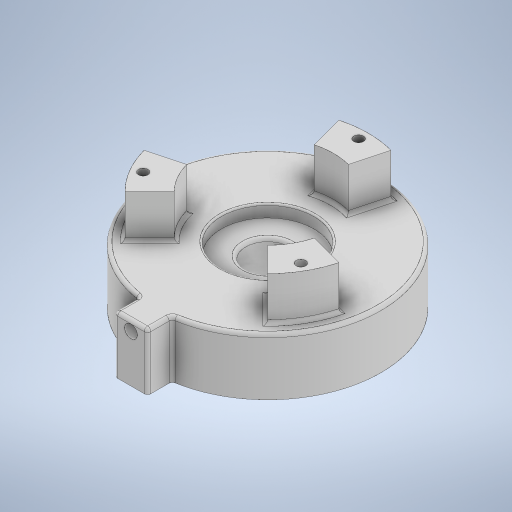
# Autodesk Inventor part: Dewar-YDS-3-Adapter
Saved by Autodesk Inventor 2023 (Build 270158000, 158)
## iProperties
Created: 2024-06-03
Part Number: Dewar-YDS-3-Adapter
Material: Generic
Document SubType Name: Modeling
Designer: incep
Density: 1 g/cm^3
Appearance: Default
Author: incep
Autodesk Inventor part; units mm, degrees
ref_plane "YZ Plane" through (0, 0, 0) normal (1, 0, 0) x (0, 1, 0)
ref_plane "XZ Plane" through (0, 0, 0) normal (0, 1, 0) x (-1, 0, 0)
sketch "Sketch1" plane through (0, 0, 0) normal (0, 1, 0) x (-1, 0, 0)
  circle A0 centre (0, 0) radius 38.75 construction
  circle A1 centre (0, 0) radius 39.25
  circle A2 centre (0, 0) radius 60.865
  circle A3 centre (0, 0) radius 60.865 construction
  dimension "d0" = 77.5
  dimension "d1" = 0.5
  dimension "d19" = 121.73
  constraints: 4 centre point, 2 coincident, 1 concentric
  measures "d0" diameter of A0
  measures "d1" radial gap between concentric circles of A0 A1
  measures "d19" diameter of A3
extrude "Extrusion1" add sketch "Sketch1" along normal blind 21
sketch "Sketch2" plane through (0, 21, 0) normal (0, 1, 0) x (1, 0, 0)
  circle A0 centre (0, 0) radius 60.865 projected
extrude "Extrusion2" add sketch "Sketch2" along normal blind 6
sketch "Sketch3" plane through (0, 27, 0) normal (0, 1, 0) x (1, 0, 0)
  circle A0 centre (0, 0) radius 12.7 construction
  circle A1 centre (0, 0) radius 13.2
  dimension "d7" = 25.4
  dimension "d8" = 0.5
  constraints: 2 centre point, 1 coincident
  measures "d7" diameter of A0
  measures "d8" radial gap between concentric circles of A0 A1
extrude "Extrusion3" cut sketch "Sketch3" against normal blind 10
sketch "Sketch4" plane through (0, 21, 0) normal (0, -1, 0) x (1, 0, 0)
  circle A0 centre (0, 0) radius 13.2 projected
  circle A1 centre (0, 0) radius 25 construction
  circle A2 centre (0, 0) radius 24.5
  dimension "d11" = 50
  dimension "d12" = 0.5
  constraints: 2 centre point, 1 coincident
  measures "d11" diameter of A1
  measures "d12" radial gap between concentric circles of A1 A2
extrude "Extrusion4" add sketch "Sketch4" along normal up to surface (21 mm away)
sketch "Sketch5" plane through (0, 27, 0) normal (0, 1, 0) x (1, 0, 0)
  circle A0 centre (0, 0) radius 60.865 projected
  circle A1 centre (0, 0) radius 27.45 construction
  circle A2 centre (0, 0) radius 27.95
  dimension "d15" = 54.9
  dimension "d16" = 0.5
  constraints: 2 centre point, 1 coincident
  measures "d15" diameter of A1
  measures "d16" radial gap between concentric circles of A1 A2
extrude "Extrusion5" add sketch "Sketch5" along normal blind 7.5
sketch "Sketch6" plane through (0, 34.5, 0) normal (0, 1, 0) x (1, 0, 0)
  circle A0 centre (0, 0) radius 27.95 construction
  circle A1 centre (0, 0) radius 55 construction
  circle A2 centre (0, 55) radius 2.9
  circle A3 centre (0, 0) radius 60.865 projected
  circle A4 centre (0, 0) radius 39.85
  line L0 (0, 0) -> (15.753, 58.7911)
  line L1 (0, 55) -> (0, 0) construction
  line L2 (0, 0) -> (-15.753, 58.7911)
  point P0 (-10.3139, 38.4921)
  point P1 (10.3139, 38.4921)
  dimension "d20" = 110
  dimension "d21" = 5.8
  dimension "d23" = 79.7
  dimension "d24" = 15
  constraints: 6 end point, 2 centre point, 2 vertical alignment, 1 coincident, 1 symmetric about line, 1 vertical, 4 other
  measures "d21" diameter of A2
  measures "d23" diameter of A4
  measures "d24" angle of L1 L0
extrude "Extrusion6" add sketch "Sketch6" along normal blind 26.1 contours L0 A4 L2 A3 picked at (9.5449, 50.3118)
pattern_circular "Circular Pattern1" count 3 over 360 about axis through (0, -10, 0) along (0, 1, 0) of "Extrusion6"
fillet "Fillet2" radius 1 1 edges at (-27.95, 34.5, 0)
sketch "Sketch7" plane through (0, 0, 0) normal (1, 0, 0) x (0, 1, 0)
  line L0 (6.175, 11.9062) -> (3, 11.9062)
  line L1 (3, 11.9062) -> (3, 15.0812)
  line L2 (3, 15.0812) -> (6.175, 15.0813)
  line L3 (6.175, 15.0813) -> (6.175, 11.9062)
  line L4 (27, -27.95) -> (27, 27.95) projected
  line L5 (-12.12, 0) -> (72.72, 0) projected
  line L6 (0, -13.2) -> (0, 13.2) projected
  line L7 (0, 24.5) -> (0, -24.5) projected
  point P0 (0, 0)
  point P1 (27, -16.2)
  point P2 (27, 16.2)
  dimension "d35" = 3.175
  dimension "d36" = 3.175
  dimension "d42" = 3
  dimension "d43" = 15.0813
  constraints: 8 end point, 2 parallel, 1 horizontal, 1 perpendicular
  measures "d35" distance of L0.start L0.end
  measures "d36" distance of L2.end L0.start
  measures "d42" distance between parallel lines of L1 L6
  measures "d43" distance from line of point (0, 0) L2
revolve "Revolution1" cut sketch "Sketch7" angle 360 about axis through (0, -10, 0) along (0, 1, 0)
sketch "Sketch9" plane through (0, 0, 0) normal (0, -1, 0) x (1, 0, 0)
  circle A0 centre (0, 0) radius 49.25
  circle A1 centre (0, 0) radius 39.25 projected
  circle A2 centre (0, 0) radius 60.865 projected
  circle A3 centre (0, 0) radius 13.2 projected
  line L0 (0, 0) -> (15.753, -58.7911)
  line L1 (0, 0) -> (0, -60.865) construction
  line L2 (0, 0) -> (-15.753, -58.7911)
  line L3 (0, 0) -> (52.7106, 30.4325) construction
  line L4 (0, 0) -> (52.7106, 30.4325)
  line L5 (0, 0) -> (58.7911, 15.753)
  point P0 (47.5718, 12.7468)
  point P1 (12.7468, -47.5718)
  dimension "d44" = 10
  dimension "d45" = 15
  dimension "d46" = 120
  dimension "d47" = 15
  constraints: 12 end point, 5 point on circle, 1 centre point, 1 coincident, 1 symmetric about line, 1 vertical
  measures "d44" radial gap between concentric circles of A0 A1
  measures "d45" angle of L0 L1
  measures "d46" angle of L1 L3
  measures "d47" angle of L5 L3
extrude "Extrusion8" cut sketch "Sketch9" against normal up to surface (34.5 mm away) contours A0 L5 A2 L0
pattern_circular "Circular Pattern2" count 3 over 360 about axis through (0, -10, 0) along (0, 1, 0) of "Extrusion8"
sketch "Sketch10" plane through (0, 0, 0) normal (0, -1, 0) x (1, 0, 0)
  circle A0 centre (0, 0) radius 68.5
  line L0 (43.0381, 43.0381) -> (34.825, 34.825) projected
  arc A1 (34.825, 34.825) -> (-34.825, 34.825) centre (0, 0) ccw projected
  line L1 (-34.825, 34.825) -> (-43.0381, 43.0381) projected
  arc A2 (-43.0381, 43.0381) -> (-58.7911, 15.753) centre (0, 0) ccw projected
  line L2 (-58.7911, 15.753) -> (-47.5718, 12.7468) projected
  arc A3 (-47.5718, 12.7468) -> (-12.7468, -47.5718) centre (0, 0) ccw projected
  line L3 (-12.7468, -47.5718) -> (-15.753, -58.7911) projected
  arc A4 (-15.753, -58.7911) -> (15.753, -58.7911) centre (0, 0) ccw projected
  line L4 (15.753, -58.7911) -> (12.7468, -47.5718) projected
  arc A5 (12.7468, -47.5718) -> (47.5718, 12.7468) centre (0, 0) ccw projected
  line L5 (47.5718, 12.7468) -> (58.7911, 15.753) projected
  arc A6 (58.7911, 15.753) -> (43.0381, 43.0381) centre (0, 0) ccw projected
  circle A7 centre (0, 0) radius 39.25 projected
  dimension "d53" = 137
  constraints: 1 centre point, 1 coincident
  measures "d53" diameter of A0
extrude "Extrusion9" add sketch "Sketch10" against normal blind 2 contours A0
sketch "Sketch11" plane through (0, 0, 0) normal (1, 0, 0) x (0, 1, 0)
  point P0 (0, 0)
ref_plane "Work Plane2" through (0, 0, 30) normal (0, 0, 1) x (1, 0, 0)
sketch "Sketch13" plane through (0, 0, 30) normal (0, 0, 1) x (1, 0, 0)
  line L0 (24.5, 21) -> (-24.5, 21) projected
  line L1 (-39.25, 21) -> (39.25, 21) projected
  circle A0 centre (0, 20.25) radius 0.75
  point P0 (0, 0)
  dimension "d57" = 1.5
  constraints: 1 centre point, 1 tangent, 1 vertical alignment
  measures "d57" diameter of A0
extrude "Extrusion10" cut sketch "Sketch13" along normal up to surface round surface about axis through (0, 0, 0) along (0, 1, 0) radius 49.25 far side no
pattern_circular "Circular Pattern3" count 3 over 360 about axis through (0, -10, 0) along (0, 1, 0) of "Extrusion10"
sketch "Sketch14" plane through (0, 2, 0) normal (0, 1, 0) x (1, 0, 0)
  circle A0 centre (0, 0) radius 68.5 projected
  circle A1 centre (0, 0) radius 66.5
  dimension "d63" = 2
  constraints: 1 centre point
  measures "d63" radial gap between concentric circles of A0 A1
extrude "Extrusion11" add sketch "Sketch14" along normal up to surface (32.5 mm away)
sketch "Sketch15" plane through (0, 34.5, 0) normal (0, 1, 0) x (1, 0, 0)
  line L0 (-10, -66.5) -> (10, -66.5)
  line L1 (10, -66.5) -> (10, -82.5)
  line L2 (10, -82.5) -> (-10, -82.5)
  line L3 (-10, -82.5) -> (-10, -66.5)
  line L4 (-4.8377, -68.5) -> (5.0753, -68.5) construction
  circle A0 centre (0, 0) radius 68.5 construction
  arc A1 (-10, -67.7661) -> (10, -67.7661) centre (0, 0) ccw
  point P0 (0, -66.5)
  dimension "d66" = 20
  dimension "d68" = 14
  dimension "d69" = 2
  constraints: 10 end point, 2 horizontal, 2 parallel, 2 point on circle, 2 point on line, 1 centre point, 1 coincident, 1 midpoint, 1 perpendicular, 1 tangent, 1 vertical alignment
  measures "d66" distance of L0.start L0.end
  measures "d68" distance between parallel lines of L2 L4
  measures "d69" distance between parallel lines of L0 L4
extrude "Extrusion12" add sketch "Sketch15" against normal up to surface (34.5 mm away) contours A1 L1 L2 L3
sketch "Sketch16" plane through (-10, 34.5, 82.5) normal (0, 0, 1) x (1, 0, 0)
  line L0 (0, 0) -> (20, 0) projected
  line L1 (4.7437, -2) -> (12.7281, -2) construction
  circle A0 centre (10, -5.85) radius 3.85
  point P0 (10, -34.5)
  point P1 (10, 0)
  dimension "d72" = 2
  dimension "d73" = 7.7
  constraints: 2 end point, 1 centre point, 1 horizontal, 1 midpoint, 1 tangent, 1 vertical alignment
  measures "d72" distance between parallel lines of L0 L1
  measures "d73" diameter of A0
extrude "Extrusion13" cut sketch "Sketch16" against normal blind 17
ref_plane "Work Plane3" through (0, 0, -68.5) normal (0, 0, 1) x (1, 0, 0)
sketch "Sketch18" plane through (0, 0, -68.5) normal (0, 0, 1) x (1, 0, 0)
  line L0 (-10, 0) -> (10, 0) projected
  line L1 (10, 0) -> (-10, 0) projected
  line L2 (-39.25, 0) -> (39.25, 0) projected
  line L3 (66.5, 2) -> (-66.5, 2) construction
  line L4 (43.0381, 2) -> (58.7911, 2) construction
  line L5 (34.825, 2) -> (43.0381, 2) construction
  line L6 (-34.825, 2) -> (34.825, 2) construction
  line L7 (-43.0381, 2) -> (-34.825, 2) construction
  line L8 (-58.7911, 2) -> (-43.0381, 2) construction
  line L9 (-47.5718, 2) -> (-58.7911, 2) construction
  line L10 (-12.7468, 2) -> (-47.5718, 2) construction
  line L11 (-15.753, 2) -> (-12.7468, 2) construction
  line L12 (15.753, 2) -> (-15.753, 2) construction
  line L13 (12.7468, 2) -> (15.753, 2) construction
  line L14 (47.5718, 2) -> (12.7468, 2) construction
  line L15 (58.7911, 2) -> (47.5718, 2) construction
  circle A0 centre (0, 3.5) radius 1.5
  point P0 (0, 0)
  point P1 (0, 0)
  dimension "d78" = 3
  constraints: 1 centre point, 1 midpoint, 1 tangent, 1 vertical alignment
  measures "d78" diameter of A0
extrude "Extrusion14" cut sketch "Sketch18" along normal blind 3
sketch "Sketch19" plane through (0, 34.5, 0) normal (0, 1, 0) x (1, 0, 0)
  arc A0 (-34.825, -34.825) -> (34.825, -34.825) centre (0, 0) ccw projected
  line L0 (34.825, -34.825) -> (28.1782, -28.1782) projected
  arc A1 (28.1782, -28.1782) -> (38.4921, -10.3139) centre (0, 0) ccw projected
  line L1 (38.4921, -10.3139) -> (47.5718, -12.7468) projected
  arc A2 (47.5718, -12.7468) -> (12.7468, 47.5718) centre (0, 0) ccw projected
  line L2 (12.7468, 47.5718) -> (10.3139, 38.4921) projected
  arc A3 (10.3139, 38.4921) -> (-10.3139, 38.4921) centre (0, 0) ccw projected
  line L3 (-10.3139, 38.4921) -> (-12.7468, 47.5718) projected
  arc A4 (-12.7468, 47.5718) -> (-47.5718, -12.7468) centre (0, 0) ccw projected
  line L4 (-47.5718, -12.7468) -> (-38.4921, -10.3139) projected
  arc A5 (-38.4921, -10.3139) -> (-28.1782, -28.1782) centre (0, 0) ccw projected
  line L5 (-28.1782, -28.1782) -> (-34.825, -34.825) projected
  circle A6 centre (0, 0) radius 28.95 projected
  arc A7 (10, -67.7661) -> (-10, -67.7661) centre (0, 0) ccw projected
  arc A8 (10.3139, 38.4921) -> (-10.3139, 38.4921) centre (0, 0) ccw projected
  line L6 (10.3139, 38.4921) -> (15.753, 58.7911) projected
  arc A9 (15.753, 58.7911) -> (-15.753, 58.7911) centre (0, 0) ccw projected
  line L7 (-15.753, 58.7911) -> (-10.3139, 38.4921) projected
  circle A10 centre (0, 55) radius 2.9 projected
  arc A11 (28.1782, -28.1782) -> (38.4921, -10.3139) centre (0, 0) ccw projected
  line L8 (28.1782, -28.1782) -> (43.0381, -43.0381) projected
  arc A12 (43.0381, -43.0381) -> (58.7911, -15.753) centre (0, 0) ccw projected
  line L9 (58.7911, -15.753) -> (38.4921, -10.3139) projected
  circle A13 centre (47.6314, -27.5) radius 2.9 projected
  arc A14 (-38.4921, -10.3139) -> (-28.1782, -28.1782) centre (0, 0) ccw projected
  line L10 (-38.4921, -10.3139) -> (-58.7911, -15.753) projected
  arc A15 (-58.7911, -15.753) -> (-43.0381, -43.0381) centre (0, 0) ccw projected
  line L11 (-43.0381, -43.0381) -> (-28.1782, -28.1782) projected
  circle A16 centre (-47.6314, -27.5) radius 2.9 projected
  circle A17 centre (0, 0) radius 66.5 projected
  point P0 (12.7468, 47.5718)
  point P1 (34.825, -34.825)
  point P2 (-47.5718, -12.7468)
extrude "Extrusion15" add sketch "Sketch19" against normal blind 2 contours A17
fillet "Fillet3" radius 2 20 edges at (0, 34.5, -68.5) (-10, 34.5, 75.1331) (0, 34.5, 82.5) (10, 34.5, 75.1331) (-35.6081, 34.5, 35.6081) (-52.7106, 34.5, 30.4325) (-48.6416, 34.5, 13.0335) (-34.5111, 34.5, 19.925) (35.6081, 34.5, 35.6081) (52.7106, 34.5, 30.4325) (48.6416, 34.5, 13.0335) (34.5111, 34.5, 19.925) (13.0335, 34.5, -48.6416) (0, 34.5, -60.865) (0, 34.5, -39.85) (-13.0335, 34.5, -48.6416) (10, 17.25, 67.7661) (10, 17.25, 82.5) (-10, 17.25, 82.5) (-10, 17.25, 67.7661)
fillet "Fillet4" radius 2 1 edges at (-13.2, 27, 0)
body "Solid1"
